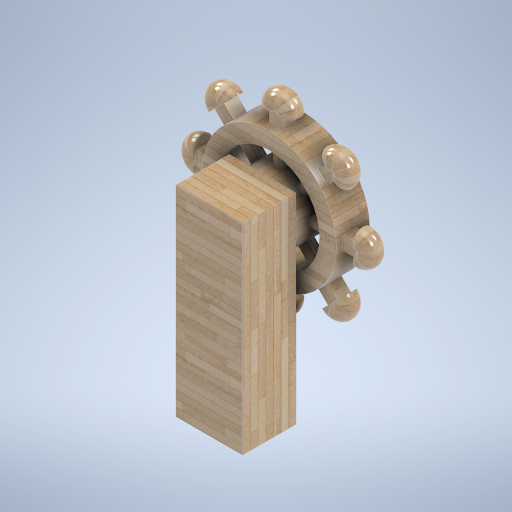
# Autodesk Inventor part: Project Wheel
Saved by Autodesk Inventor 2024 (Build 280153000, 153)
## iProperties
Created: 2023-10-18
Part Number: Project Wheel
Material: Wood (Maple)
Document SubType Name: Modeling
Designer: dde
Density: 0.67 g/cm^3
Appearance: Natural Maple - Glossy Dark Tint
Author: dde
Autodesk Inventor part; units mm, degrees
ref_plane "YZ Plane" through (0, 0, 0) normal (1, 0, 0) x (0, 1, 0)
sketch "Sketch1" plane through (0, 0, 0) normal (0, 0, 1) x (1, 0, 0)
  line L0 (0, 0) -> (500, 0)
  line L1 (500, 0) -> (500, 1500)
  line L2 (500, 1500) -> (0, 1500)
  line L3 (0, 1500) -> (0, 0)
  dimension "d0" = 500
  dimension "d1" = 1500
  constraints: 8 end point, 2 parallel, 1 horizontal, 1 perpendicular
  measures "d0" distance of L2.end L1.end
  measures "d1" distance of L1.end L0.end
extrude "Extrusion1" add sketch "Sketch1" along normal blind 400
sketch "Sketch2" plane through (0, 0, 0) normal (0, 0, 1) x (1, 0, 0)
  circle A0 centre (250, 1250) radius 250
  line L0 (500, 1500) -> (0, 1500) projected
  line L1 (0, 1500) -> (0, 0) projected
  dimension "d4" = 500
  dimension "d5" = 250
  dimension "d6" = 250
  constraints: 1 centre point
  measures "d4" diameter of A0
  measures "d5" distance from line of L0 A0.centre
  measures "d6" distance from line of L1 A0.centre
extrude "Extrusion2" add sketch "Sketch2" along normal mid plane 600 contours A0
sketch "Sketch4" plane through (0, 0, 0) normal (1, 0, 0) x (0, 1, 0)
  circle A0 centre (1250, -150) radius 50
  line L0 (1500, 0) -> (1250, 0) projected
  point P0 (0, 0)
  dimension "d15" = 100
  dimension "d16" = 150
  dimension "d17" = 250
  constraints: 1 centre point
  measures "d15" diameter of A0
  measures "d16" distance from line of L0 A0.centre
  measures "d17" horizontal distance of L0.start A0.centre
extrude "Extrusion4" add sketch "Sketch4" against normal blind 250
pattern_circular "Circular Pattern2" count 8 over 360 about axis through (250, 1250, 0) along (0, 0, 1) of "Extrusion4"
ref_plane "Work Plane1" through (0, 0, -300) normal (0, 0, 1) x (1, 0, 0)
sketch "Sketch5" plane through (0, 0, -300) normal (0, 0, 1) x (1, 0, 0)
  arc A0 (500, 1250) -> (250, 1500) centre (250, 1250) ccw projected
  circle A1 centre (250, 1250) radius 375
  circle A2 centre (250, 1250) radius 500
  point P0 (0, 0)
  dimension "d24" = 750
  dimension "d25" = 1000
  constraints: 2 centre point, 2 coincident
  measures "d24" diameter of A1
  measures "d25" diameter of A2
extrude "Extrusion5" add sketch "Sketch5" along normal blind 250
ref_plane "Work Plane2" through (0, 1250, 0) normal (0, 1, 0) x (-1, 0, 0)
sketch "Sketch6" plane through (0, 1250, 0) normal (0, 1, 0) x (-1, 0, 0)
  line L0 (250, -200) -> (250, -100) projected
  line L1 (250, -200) -> (350, -200)
  line L2 (350, -200) -> (350, -100)
  line L3 (350, -100) -> (250, -100)
  line L4 (250, -100) -> (250, -200)
  arc A0 (350, -200) -> (350, -100) centre (405.5666, -150) ccw
  point P0 (0, 0)
  dimension "d29" = 100
  dimension "d30" = 100
  constraints: 8 end point, 2 parallel, 2 point on circle, 1 centre point, 1 horizontal, 1 perpendicular
  measures "d29" distance of L3.end L2.end
  measures "d30" distance of L2.end L1.end
extrude "Extrusion6" add sketch "Sketch6" along normal mid plane 100 contours L0 L3 L2 L1
revolve "Revolution1" add sketch "Sketch6" angle 180 mid plane about axis through (-350, 1250, -200) along (0, 0, 1) contours L2 A0
pattern_circular "Circular Pattern3" count 8 over 360 about axis through (250, 1250, -300) along (0, 0, 1) of "Extrusion6", "Revolution1"
body "Solid1"
